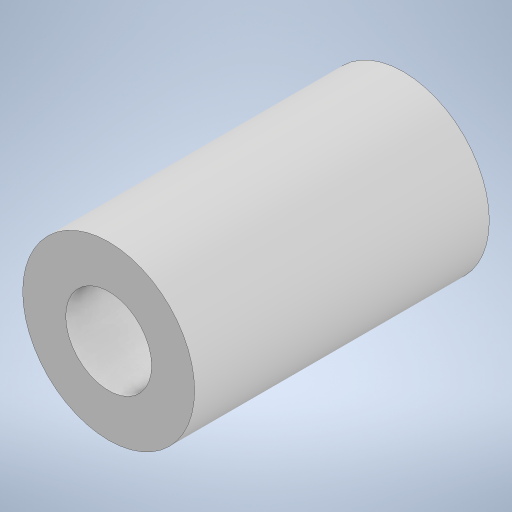
# Autodesk Inventor part: CircularStandOff
Saved by Autodesk Inventor 2023 (Build 270158000, 158)
## iProperties
Created: 2023-06-03
Part Number: CircularStandOff
Material: Ogólny
Document SubType Name: Modeling
Designer: Kamil
Density: 1 g/cm^3
Appearance: Domyślna
Author: Kamil
Autodesk Inventor part; units mm, degrees
ref_plane "YZ Plane" through (0, 0, 0) normal (1, 0, 0) x (0, 1, 0)
ref_plane "XZ Plane" through (0, 0, 0) normal (0, 1, 0) x (-1, 0, 0)
ref_plane "XY Plane" through (0, 0, 0) normal (0, 0, 1) x (1, 0, 0)
sketch "Szkic1" plane through (0, 0, 0) normal (0, 0, 1) x (1, 0, 0)
  circle A0 centre (2.056, -2.83) radius 1.75
  circle A1 centre (2.0547, -2.8314) radius 3.5
  point P0 (0, 0)
  point P1 (2.0561, -2.83)
  dimension "d2" = 7
  dimension "d3" = 3.5
  constraints: 2 centre point
  measures "d2" diameter of A1
  measures "d3" diameter of A0
extrude "Wyciągnięcie proste1" add sketch "Szkic1" along normal blind 12
